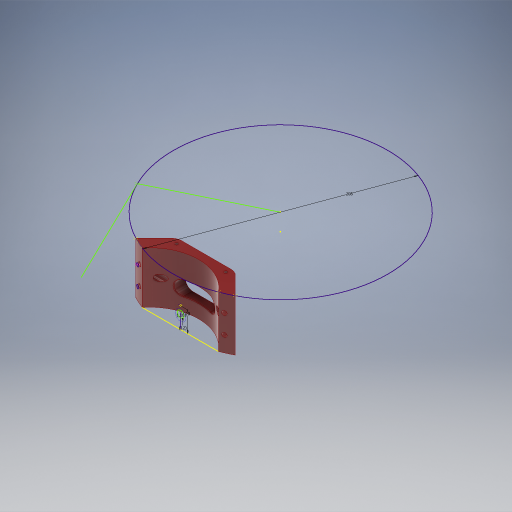
# Autodesk Inventor part: catch_v2
Saved by Autodesk Inventor 2023 (Build 270158000, 158)
## iProperties
Created: 2024-11-02
Part Number: catch_v2
Material: Полиэтилен, низкая плотность
Document SubType Name: Sheet Metal
Designer: Ivan
Density: 0.579707 g/cm^3
Appearance: Типовые
Mass: 30 g
Surface Area: 146.87 cm^2
Volume: 51.7503 cm^3
Sheet Metal Rule: По умолчанию
Author: Ivan
Autodesk Inventor part; units mm, degrees
ref_plane "YZ Plane" through (0, 0, 0) normal (1, 0, 0) x (0, 1, 0)
ref_plane "XZ Plane" through (0, 0, 0) normal (0, 1, 0) x (-1, 0, 0)
ref_plane "XY Plane" through (0, 0, 0) normal (0, 0, 1) x (1, 0, 0)
derived "floor_v2.ipt"
sketch "Эскиз2" plane through (0, 0, 0) normal (0, 1, 0) x (1, 0, 0)
  circle A0 centre (0, 0) radius 107.5
  circle A1 centre (0, 0) radius 104
  line L0 (0, 0) -> (104, 0) construction
  line L1 (0, 0) -> (0, -104) construction
  line L2 (0, 0) -> (-104, 0) construction
  line L3 (0, 0) -> (0, 104) construction
  line L4 (104, 0) -> (0, -104) construction
  line L5 (0, 104) -> (-104, 0) construction
  line L6 (0, -104) -> (-104, 0) construction
  line L7 (104, 0) -> (0, 104) construction
  line L8 (0, 0) -> (-73.5391, -73.5391) construction
  line L9 (0, 0) -> (73.5391, -73.5391) construction
  line L10 (0, 0) -> (73.5391, 73.5391) construction
  line L11 (0, 0) -> (-73.5391, 73.5391) construction
  line L12 (-38.4471, -82.2877) -> (-82.2877, -38.4471)
  line L13 (-38.4471, -82.2877) -> (-48.2758, -92.1165)
  line L14 (-82.2877, -38.4471) -> (-92.1165, -48.2758)
  line L15 (92.1165, -48.2758) -> (82.2877, -38.4471)
  line L16 (82.2877, -38.4471) -> (38.4471, -82.2877)
  line L17 (38.4471, -82.2877) -> (48.2758, -92.1165)
  line L18 (48.2758, 92.1165) -> (38.4471, 82.2877)
  line L19 (38.4471, 82.2877) -> (82.2877, 38.4471)
  line L20 (82.2877, 38.4471) -> (92.1165, 48.2758)
  line L21 (-48.2758, 92.1165) -> (-38.4471, 82.2877)
  line L22 (-38.4471, 82.2877) -> (-82.2877, 38.4471)
  line L23 (-82.2877, 38.4471) -> (-92.1165, 48.2758)
  line L24 (0, -107.5) -> (0, -79.5) construction
  circle A2 centre (0, -116.5) radius 37 construction
  circle A3 centre (0, -127) radius 47.5
  line L25 (0, 107.5) -> (0, 79.5) construction
  circle A4 centre (0, 127) radius 47.5
  line L26 (-92.1165, 48.2758) -> (-94.7051, 50.8645)
  line L27 (-48.2758, 92.1165) -> (-50.8645, 94.7051)
  line L28 (48.2758, 92.1165) -> (50.8645, 94.7051)
  line L29 (92.1165, 48.2758) -> (94.7051, 50.8645)
  line L30 (92.1165, -48.2758) -> (94.7051, -50.8645)
  line L31 (48.2758, -92.1165) -> (50.8645, -94.7051)
  line L32 (-92.1165, -48.2758) -> (-94.7051, -50.8645)
  line L33 (-48.2758, -92.1165) -> (-50.8645, -94.7051)
  point P0 (-52, -52)
  point P1 (-52, 52)
  point P2 (52, 52)
  point P3 (52, -52)
  point P4 (-60.3674, -60.3674)
  point P5 (60.3674, -60.3674)
  point P6 (60.3674, 60.3674)
  point P7 (-60.3674, 60.3674)
  point P8 (-36.9892, -97.1998)
  point P9 (36.9892, -97.1998)
  point P10 (36.9892, 97.1998)
  point P11 (-36.9892, 97.1998)
sketch "Эскиз3" plane through (0, 2, 0) normal (0, -1, 0) x (-1, 0, 0)
  line L0 (33.8509, 77.6915) -> (77.6915, 33.8509) construction
  line L1 (55.7712, 55.7712) -> (0, 0) construction
  line L2 (44.4575, 67.0849) -> (67.0849, 44.4575) construction
  circle A0 centre (44.4575, 67.0849) radius 1.5
  circle A1 centre (67.0849, 44.4575) radius 1.5
  line L3 (28.3991, 51.0265) -> (51.0265, 28.3991) construction
  circle A2 centre (28.3991, 51.0265) radius 1.5
  circle A3 centre (51.0265, 28.3991) radius 1.5
  line L4 (44.4575, -67.0849) -> (67.0849, -44.4575) construction
  line L5 (28.3991, -51.0265) -> (51.0265, -28.3991) construction
  line L6 (55.7712, -55.7712) -> (0, 0) construction
  line L7 (-55.7712, -55.7712) -> (0, 0) construction
  line L8 (-28.3991, -51.0265) -> (-51.0265, -28.3991) construction
  line L9 (-44.4575, -67.0849) -> (-67.0849, -44.4575) construction
  line L10 (-55.7712, 55.7712) -> (0, 0) construction
  line L11 (-51.0265, 28.3991) -> (-28.3991, 51.0265) construction
  line L12 (-67.0849, 44.4575) -> (-44.4575, 67.0849) construction
  circle A4 centre (-44.4575, 67.0849) radius 1.5
  circle A5 centre (-67.0849, 44.4575) radius 1.5
  circle A6 centre (-28.3991, 51.0265) radius 1.5
  circle A7 centre (-51.0265, 28.3991) radius 1.5
  circle A8 centre (-44.4575, -67.0849) radius 1.5
  circle A9 centre (-67.0849, -44.4575) radius 1.5
  circle A10 centre (-51.0265, -28.3991) radius 1.5
  circle A11 centre (-28.3991, -51.0265) radius 1.5
  circle A12 centre (44.4575, -67.0849) radius 1.5
  circle A13 centre (28.3991, -51.0265) radius 1.5
  circle A14 centre (51.0265, -28.3991) radius 1.5
  circle A15 centre (67.0849, -44.4575) radius 1.5
  line L13 (-38.4471, -82.2877) -> (-82.2877, -38.4471)
  line L14 (82.2877, -38.4471) -> (38.4471, -82.2877)
  line L15 (38.4471, 82.2877) -> (82.2877, 38.4471)
  line L16 (-82.2877, 38.4471) -> (-38.4471, 82.2877)
  line L17 (82.2877, 38.4471) -> (92.1165, 48.2758)
  point P0 (39.7128, 39.7128)
  point P1 (-39.7128, -39.7128)
  point P2 (39.7128, -39.7128)
  point P3 (-39.7128, 39.7128)
  point P4 (-40.1306, -40.1306)
sketch "Эскиз6" plane through (0, 2, 0) normal (0, -1, 0) x (-1, 0, 0)
  arc A0 (36.9892, -97.1998) -> (-36.9892, -97.1998) centre (0, -127) ccw
  arc A1 (-36.9892, 97.1998) -> (36.9892, 97.1998) centre (0, 127) ccw
  point P0 (-0.0301, 154.5629)
  point P1 (-0.0412, -154.5628)
sketch "Эскиз8" plane through (0, 2, 0) normal (0, 1, 0) x (1, 0, 0)
  arc A0 (-48.2758, -92.1165) -> (-36.9892, -97.1998) centre (0, 0) ccw
  arc A1 (36.9892, -97.1998) -> (48.2758, -92.1165) centre (0, 0) ccw
  arc A2 (36.9892, -97.1998) -> (-36.9892, -97.1998) centre (0, -127) ccw
  circle A3 centre (0, -127) radius 55.4164 construction
  circle A4 centre (-23.8556, -76.9811) radius 1.5
  circle A5 centre (23.8556, -76.9811) radius 1.5
  circle A6 centre (-28.3991, -51.0265) radius 1.5 construction
  circle A7 centre (-51.0265, -28.3991) radius 1.5 construction
  circle A8 centre (-67.0849, -44.4575) radius 1.5 construction
  circle A9 centre (-44.4575, -67.0849) radius 1.5 construction
  circle A10 centre (-51.0265, -28.3991) radius 1.5 construction
  line L0 (-51.0265, -28.3991) -> (-28.3991, -51.0265) construction
  line L1 (-67.0849, -44.4575) -> (-44.4575, -67.0849) construction
  line L2 (-55.7712, -55.7712) -> (-39.7128, -39.7128) construction
  line L3 (-50.4184, -50.4184) -> (-23.8556, -76.9811) construction
  circle A11 centre (67.0849, -44.4575) radius 1.5 construction
  circle A12 centre (44.4575, -67.0849) radius 1.5 construction
  line L4 (44.4575, -67.0849) -> (67.0849, -44.4575) construction
  arc A13 (-92.1165, 48.2758) -> (-92.1165, -48.2758) centre (0, 0) ccw construction
  line L5 (-104, 0) -> (104, 0) construction
  arc A14 (92.1165, -48.2758) -> (92.1165, 48.2758) centre (0, 0) ccw construction
  circle A15 centre (-23.8556, 76.9811) radius 1.5
  circle A16 centre (23.8556, 76.9811) radius 1.5
  point P0 (-44.5136, -93.9922)
  point P1 (-104, 0)
sketch "Эскиз5" plane through (0, 0, 0) normal (0, 1, 0) x (-1, 0, 0)
  arc A0 (-36.9892, 97.1998) -> (36.9892, 97.1998) centre (0, 127) ccw projected
  circle A1 centre (0, 0) radius 104 projected
  line L0 (38.4471, 82.2877) -> (48.2758, 92.1165) projected
  line L1 (-38.4471, 82.2877) -> (-48.2758, 92.1165) projected
  line L2 (38.4471, 82.2877) -> (28.1405, 71.9811)
  line L3 (-38.4471, 82.2877) -> (-28.1405, 71.9811)
  line L4 (28.1405, 71.9811) -> (-28.1405, 71.9811)
  line L5 (82.2877, 38.4471) -> (38.4471, 82.2877) projected
  circle A2 centre (23.8556, 76.9811) radius 1.5 projected
  circle A3 centre (-23.8556, 76.9811) radius 1.5 projected
  circle A4 centre (23.8556, 76.9811) radius 5 construction
  circle A5 centre (-23.8556, 76.9811) radius 5 construction
  dimension "d3" = 10
  constraints: 6 end point, 2 centre point, 2 coincident, 2 collinear, 2 tangent, 1 horizontal, 1 perpendicular
  measures "d3" diameter of A5
extrude "Выдавливание1" add sketch "Эскиз5" along normal blind 50 contours A0 A1 L0 L2 L4 L3 L1 | A2 | A3
ref_plane "РабПлоскость2" through (0, 0, 43.8406) normal (-1, 0, 0) x (0, 1, 0)
sketch "Эскиз9" plane through (0, 50, 0) normal (0, 1, 0) x (1, 0, 0)
  circle A0 centre (-23.8556, -76.9811) radius 1.5 projected
  circle A1 centre (23.8556, -76.9811) radius 1.5 projected
  point P0 (0, 0)
hole "Отверстие1" at (-23.8556, 50, 76.9811) at (23.8556, 50, 76.9811) direction (0, -1, 0) diameter 3.2 depth 7
hole "Отверстие2" at (-23.8556, 0, 76.9811) at (23.8556, 0, 76.9811) direction (0, 1, 0) diameter 3.2 depth 7
fillet "Сопряжение1" radius 10 2 edges at (-28.1405, 25, 71.9811) (28.1405, 25, 71.9811)
ref_plane "РабПлоскость1" through (-36.9892, 50, 97.1998) normal (-1, 0, 0) x (0, 1, 0)
sketch "Эскиз10" plane through (-36.9892, 50, 97.1998) normal (-1, 0, 0) x (0, 1, 0)
  line L0 (-50, 0) -> (0, 0) projected
  line L1 (-25, 0) -> (-25, -14.2479)
  circle A0 centre (-25, 8.49) radius 3.1
  line L2 (0, 17.6998) -> (0, 0) projected
  line L3 (0, 17.6998) -> (-25, 17.6998)
  line L4 (0, 17.6998) -> (-50, 17.6998) projected
  point P0 (-50, 97.1998)
  dimension "d21" = 6.2
  dimension "d54" = 8.49
  constraints: 4 end point, 2 midpoint, 2 point on line, 1 centre point, 1 perpendicular
  measures "d21" diameter of A0
  measures "d54" distance from line of L0 A0.centre
extrude "Выдавливание2" cut sketch "Эскиз10" along normal through all both and the other way through all
mirror "Зеркальное отражение1" about plane through (0, 0, 43.8406) normal (-1, 0, 0) of "Выдавливание2"
ref_plane "РабПлоскость3" through (0, 25, 0) normal (0, 1, 0) x (1, 0, 0)
sketch "Эскиз13" plane through (48.2758, 0, 92.1165) normal (0.7071068, 0, -0.7071068) x (-0.7071068, 0, -0.7071068)
  line L0 (-186.6107, 25) -> (379.5577, 25) projected
  line L1 (24.3335, 50) -> (24.3335, 0) projected
  point P0 (99.2724, 0)
sketch "Эскиз17" plane through (0, 50, 0) normal (0, 1, 0) x (1, 0, 0)
  line L0 (-31.0695, -74.9101) -> (-48.2758, -92.1165) projected
  arc A0 (-48.2758, -92.1165) -> (-36.9892, -97.1998) centre (0, 0) ccw projected
  line L1 (-40.9045, -84.7452) -> (-40.9045, -95.6181)
  line L2 (-36.9892, -79.5) -> (-36.9892, -97.1998) projected
  arc A1 (36.9892, -97.1998) -> (-36.9892, -97.1998) centre (0, -127) ccw projected
  line L3 (-24.2555, -86.1598) -> (-42.3192, -86.1598) projected
  line L4 (-31.9045, -91.8098) -> (-47.9692, -91.8098) projected
  dimension "d55" = 9
  constraints: 2 end point, 1 parallel, 1 point on circle, 1 point on line
  measures "d55" distance from line of L1 L4.start
ref_plane "РабПлоскость5" through (-40.9045, 50, 95.6181) normal (-1, 0, 0) x (0, 1, 0)
sketch "Эскиз18" plane through (-40.9045, 50, 95.6181) normal (-1, 0, 0) x (0, 1, 0)
  circle A0 centre (-25, 6.9083) radius 3.1 projected
  circle A1 centre (-25, 6.9083) radius 3.1
  point P0 (-50, 95.6181)
  dimension "d56" = 6.2
  constraints: 2 coincident, 1 centre point
  measures "d56" diameter of A1
extrude "Выдавливание7" cut sketch "Эскиз18" along normal blind 13
mirror "Зеркальное отражение3" about plane through (0, 0, 43.8406) normal (-1, 0, 0) of "Выдавливание7"
ref_plane "РабПлоскость7" through (36.9892, 50, 97.1998) normal (-0.6749966, 0, -0.7378208) x (-0.7378208, 0, 0.6749966)
ref_plane "РабПлоскость6" through (93.533, -2, 45.4705) normal (-0.6749966, 0, -0.7378208) x (-0.7378208, 0, 0.6749966)
sketch "Эскиз19" plane through (36.9892, 50, 97.1998) normal (-0.6749966, 0, -0.7378208) x (-0.7378208, 0, 0.6749966)
  spline S0 degree 3 poles (-7.7154, -10.575) (-7.7154, -10.6506) (-7.71, -10.7286) (-7.6802, -10.9332) (-7.6461, -11.0604) (-7.5316, -11.3409) (-7.4453, -11.4844) (-7.2515, -11.7106) (-7.1586, -11.7978) (-6.897, -11.9868) (-6.7118, -12.075) (-6.3289, -12.1741) (-6.1042, -12.1918) (-5.7271, -12.1319) (-5.5774, -12.0862) (-5.2959, -11.9511) (-5.167, -11.8652) (-4.8829, -11.6031) (-4.7406, -11.4053) (-4.5272, -10.8834) (-4.4982, -10.5576) (-4.6133, -10.0143) (-4.7143, -9.7949) (-4.9564, -9.4713) (-5.0835, -9.3525) (-5.3442, -9.1705) (-5.4898, -9.0986) (-5.9017, -8.9666) (-6.1741, -8.9581) (-6.6389, -9.0429) (-6.8486, -9.1334) (-7.1761, -9.3613) (-7.2993, -9.4844) (-7.4685, -9.7101) (-7.5294, -9.8144) (-7.6283, -10.0387) (-7.6645, -10.1561) (-7.7063, -10.3754) (-7.7154, -10.4772) (-7.7154, -10.575) knots 0 0 0 0 0.030068 0.030068 0.078176 0.078176 0.140718 0.140718 0.183173 0.183173 0.246087 0.246087 0.309229 0.309229 0.349946 0.349946 0.390663 0.390663 0.445235 0.445235 0.518423 0.518423 0.571305 0.571305 0.612987 0.612987 0.654495 0.654495 0.727263 0.727263 0.799075 0.799075 0.857025 0.857025 0.901749 0.901749 0.946474 0.946474 0.985357 0.985357 0.985357 0.985357 weights 1 1 1 1 1 1 1 1 1 1 1 1 1 1 1 1 1 1 1 1 1 1 1 1 1 1 1 1 1 1 1 1 1 1 1 1 1 1 1 1 projected
  spline S1 degree 3 poles (-7.7154, -40.575) (-7.7154, -40.6506) (-7.71, -40.7286) (-7.6802, -40.9332) (-7.6461, -41.0604) (-7.5316, -41.3409) (-7.4453, -41.4844) (-7.2515, -41.7106) (-7.1586, -41.7978) (-6.897, -41.9868) (-6.7118, -42.075) (-6.3289, -42.1741) (-6.1042, -42.1918) (-5.7271, -42.1319) (-5.5774, -42.0862) (-5.2959, -41.9511) (-5.167, -41.8652) (-4.8829, -41.6031) (-4.7406, -41.4053) (-4.5272, -40.8834) (-4.4982, -40.5576) (-4.6133, -40.0143) (-4.7143, -39.7949) (-4.9564, -39.4713) (-5.0835, -39.3525) (-5.3442, -39.1705) (-5.4898, -39.0986) (-5.9017, -38.9666) (-6.1741, -38.9581) (-6.6389, -39.0429) (-6.8486, -39.1334) (-7.1761, -39.3613) (-7.2993, -39.4844) (-7.4685, -39.7101) (-7.5294, -39.8144) (-7.6283, -40.0387) (-7.6645, -40.1561) (-7.7063, -40.3754) (-7.7154, -40.4772) (-7.7154, -40.575) knots 0 0 0 0 0.030068 0.030068 0.078176 0.078176 0.140718 0.140718 0.183173 0.183173 0.246087 0.246087 0.309229 0.309229 0.349946 0.349946 0.390663 0.390663 0.445235 0.445235 0.518423 0.518423 0.571305 0.571305 0.612987 0.612987 0.654495 0.654495 0.727263 0.727263 0.799075 0.799075 0.857025 0.857025 0.901749 0.901749 0.946474 0.946474 0.985357 0.985357 0.985357 0.985357 weights 1 1 1 1 1 1 1 1 1 1 1 1 1 1 1 1 1 1 1 1 1 1 1 1 1 1 1 1 1 1 1 1 1 1 1 1 1 1 1 1 projected
  point P0 (-38.3182, -50)
  point P1 (-7.7154, -10.575)
  point P2 (-7.7154, -40.575)
ref_plane "РабПлоскость8" through (-36.9892, 50, 97.1998) normal (0, 0, 1) x (0, -1, 0)
sketch "Эскиз21" plane through (-36.9892, 50, 97.1998) normal (0, 0, 1) x (0, -1, 0)
  ellipse E0 centre (38, 37.1664) end of major axis (32.9, 37.1664) minor radius 5.1 construction
  line L0 (50, 0) -> (50, 73.9783) projected
  line L1 (38, 37.1664) -> (50, 37.1664)
  circle A0 centre (36.839, 37.1664) radius 3.1623
  point P0 (50, 36.9892)
  point P1 (30, 37.1664)
  dimension "d75" = 12
  dimension "d76" = 1.161
  dimension "d93" = 20
  constraints: 3 point on line, 2 end point, 1 centre point, 1 perpendicular, 3 other
  measures "d75" distance of L1.start L1.end
  measures "d76" distance of L1.start A0.centre
  measures "d93" distance from line of point (30, 37.166) L0
hole "Отверстие5" at (0.1772, 20, 97.1998) direction (0, 0, -1) diameter 13.5 end through all
sketch "Эскиз23" plane through (0, 50, 0) normal (0, 1, 0) x (1, 0, 0)
  circle A0 centre (0, 0) radius 104
  line L0 (-93.5502, -45.4353) -> (-42.0243, -151.5258)
  line L1 (-93.5502, -45.4353) -> (0, 0)
  arc A1 (-48.2758, -92.1165) -> (-36.9892, -97.1998) centre (0, 0) ccw projected
  point P0 (48.2758, -92.1165)
  point P1 (36.9892, -97.1998)
  dimension "d77" = 208
  constraints: 4 end point, 2 point on circle, 1 centre point, 1 concentric, 1 point on line, 1 tangent
  measures "d77" diameter of A0
ref_plane "РабПлоскость9" through (-41.7508, 33.5167, 97.0505) normal (0, 1, 0) x (1, 0, 0)
sketch "Эскиз24" plane through (-41.7508, 33.5167, 97.0505) normal (0, 1, 0) x (1, 0, 0)
  point P0 (41.7508, 97.0505)
  point P1 (0, 0)
ref_plane "РабПлоскость10" through (-41.7508, 33.5167, 97.0505) normal (-0.3951802, 0, 0.9186036) x (0, -1, 0)
sketch "Эскиз25" plane through (-41.7508, 33.5167, 97.0505) normal (-0.3951802, 0, 0.9186036) x (0, -1, 0)
  spline S0 degree 3 poles (-1.6, 0) (-1.6, 0.0991) (-1.5907, 0.2016) (-1.5393, 0.4672) (-1.4807, 0.6292) (-1.2922, 0.9686) (-1.154, 1.1294) (-0.8735, 1.3476) (-0.7502, 1.4203) (-0.4207, 1.5587) (-0.2036, 1.6) (0.2036, 1.6) (0.4207, 1.5587) (0.8178, 1.392) (0.9977, 1.2668) (1.321, 0.9392) (1.4676, 0.6925) (1.6159, 0.1629) (1.6205, -0.1058) (1.5045, -0.5857) (1.408, -0.7897) (1.1869, -1.0839) (1.0823, -1.1886) (0.8337, -1.3744) (0.6918, -1.4515) (0.3653, -1.569) (0.1774, -1.6) (-0.0952, -1.6) (-0.1934, -1.5914) (-0.5126, -1.5323) (-0.7306, -1.4409) (-0.9964, -1.2559) (-1.0718, -1.1917) (-1.2278, -1.0337) (-1.3094, -0.9291) (-1.4884, -0.6265) (-1.5607, -0.4119) (-1.5959, -0.1327) (-1.6, -0.0656) (-1.6, 0) knots 0.72325 0.72325 0.72325 0.72325 0.753388 0.753388 0.801609 0.801609 0.864296 0.864296 0.904063 0.904063 0.964334 0.964334 1.024605 1.024605 1.084875 1.084875 1.162686 1.162686 1.242644 1.242644 1.304846 1.304846 1.349406 1.349406 1.393966 1.393966 1.446501 1.446501 1.474685 1.474685 1.538426 1.538426 1.567042 1.567042 1.605057 1.605057 1.667632 1.667632 1.687584 1.687584 1.687584 1.687584 weights 1 1 1 1 1 1 1 1 1 1 1 1 1 1 1 1 1 1 1 1 1 1 1 1 1 1 1 1 1 1 1 1 1 1 1 1 1 1 1 1
  spline S1 degree 3 poles (16.7833, 0) (16.7833, 0.0991) (16.7927, 0.2016) (16.844, 0.4672) (16.9026, 0.6292) (17.0911, 0.9686) (17.2293, 1.1294) (17.5098, 1.3476) (17.6331, 1.4203) (17.9627, 1.5587) (18.1798, 1.6) (18.5869, 1.6) (18.804, 1.5587) (19.2011, 1.392) (19.3811, 1.2668) (19.7044, 0.9392) (19.851, 0.6925) (19.9992, 0.1629) (20.0038, -0.1058) (19.8879, -0.5857) (19.7913, -0.7897) (19.5702, -1.0839) (19.4656, -1.1886) (19.217, -1.3744) (19.0751, -1.4515) (18.7486, -1.569) (18.5608, -1.6) (18.2881, -1.6) (18.1899, -1.5914) (17.8707, -1.5323) (17.6527, -1.4409) (17.387, -1.2559) (17.3115, -1.1917) (17.1555, -1.0337) (17.074, -0.9291) (16.895, -0.6265) (16.8226, -0.4119) (16.7874, -0.1327) (16.7833, -0.0656) (16.7833, 0) knots 0.72325 0.72325 0.72325 0.72325 0.753388 0.753388 0.801609 0.801609 0.864296 0.864296 0.904063 0.904063 0.964334 0.964334 1.024605 1.024605 1.084875 1.084875 1.162686 1.162686 1.242644 1.242644 1.304846 1.304846 1.349406 1.349406 1.393966 1.393966 1.446501 1.446501 1.474685 1.474685 1.538426 1.538426 1.567042 1.567042 1.605057 1.605057 1.667632 1.667632 1.687584 1.687584 1.687584 1.687584 weights 1 1 1 1 1 1 1 1 1 1 1 1 1 1 1 1 1 1 1 1 1 1 1 1 1 1 1 1 1 1 1 1 1 1 1 1 1 1 1 1
  constraints: 4 other
sketch "Эскиз26" plane through (-41.7508, 33.5167, 97.0505) normal (-0.3951802, 0, 0.9186036) x (0, -1, 0)
  spline S0 degree 3 poles (-1.6, 0) (-1.6, 0.0991) (-1.5907, 0.2016) (-1.5393, 0.4672) (-1.4807, 0.6292) (-1.2922, 0.9686) (-1.154, 1.1294) (-0.8735, 1.3476) (-0.7502, 1.4203) (-0.4207, 1.5587) (-0.2036, 1.6) (0.2036, 1.6) (0.4207, 1.5587) (0.8178, 1.392) (0.9977, 1.2668) (1.321, 0.9392) (1.4676, 0.6925) (1.6159, 0.1629) (1.6205, -0.1058) (1.5045, -0.5857) (1.408, -0.7897) (1.1869, -1.0839) (1.0823, -1.1886) (0.8337, -1.3744) (0.6918, -1.4515) (0.3653, -1.569) (0.1774, -1.6) (-0.0952, -1.6) (-0.1934, -1.5914) (-0.5126, -1.5323) (-0.7306, -1.4409) (-0.9964, -1.2559) (-1.0718, -1.1917) (-1.2278, -1.0337) (-1.3094, -0.9291) (-1.4884, -0.6265) (-1.5607, -0.4119) (-1.5959, -0.1327) (-1.6, -0.0656) (-1.6, 0) knots 0.72325 0.72325 0.72325 0.72325 0.753388 0.753388 0.801609 0.801609 0.864296 0.864296 0.904063 0.904063 0.964334 0.964334 1.024605 1.024605 1.084875 1.084875 1.162686 1.162686 1.242644 1.242644 1.304846 1.304846 1.349406 1.349406 1.393966 1.393966 1.446501 1.446501 1.474685 1.474685 1.538426 1.538426 1.567042 1.567042 1.605057 1.605057 1.667632 1.667632 1.687584 1.687584 1.687584 1.687584 weights 1 1 1 1 1 1 1 1 1 1 1 1 1 1 1 1 1 1 1 1 1 1 1 1 1 1 1 1 1 1 1 1 1 1 1 1 1 1 1 1 construction
  circle A0 centre (0, 0) radius 2
  line L0 (33.5167, 4.4331) -> (-16.4833, 4.4331) projected
  line L1 (8.5167, 4.4331) -> (8.5167, -8) construction
  line L2 (-16.4833, -67.9804) -> (-16.4833, 21.2763) projected
  line L3 (33.5167, 4.4331) -> (33.5167, -7.9438) projected
  spline S1 degree 3 poles (16.7833, 0) (16.7833, 0.0991) (16.7927, 0.2016) (16.844, 0.4672) (16.9026, 0.6292) (17.0911, 0.9686) (17.2293, 1.1294) (17.5098, 1.3476) (17.6331, 1.4203) (17.9627, 1.5587) (18.1798, 1.6) (18.5869, 1.6) (18.804, 1.5587) (19.2011, 1.392) (19.3811, 1.2668) (19.7044, 0.9392) (19.851, 0.6925) (19.9992, 0.1629) (20.0038, -0.1058) (19.8879, -0.5857) (19.7913, -0.7897) (19.5702, -1.0839) (19.4656, -1.1886) (19.217, -1.3744) (19.0751, -1.4515) (18.7486, -1.569) (18.5608, -1.6) (18.2881, -1.6) (18.1899, -1.5914) (17.8707, -1.5323) (17.6527, -1.4409) (17.387, -1.2559) (17.3115, -1.1917) (17.1555, -1.0337) (17.074, -0.9291) (16.895, -0.6265) (16.8226, -0.4119) (16.7874, -0.1327) (16.7833, -0.0656) (16.7833, 0) knots 0.72325 0.72325 0.72325 0.72325 0.753388 0.753388 0.801609 0.801609 0.864296 0.864296 0.904063 0.904063 0.964334 0.964334 1.024605 1.024605 1.084875 1.084875 1.162686 1.162686 1.242644 1.242644 1.304846 1.304846 1.349406 1.349406 1.393966 1.393966 1.446501 1.446501 1.474685 1.474685 1.538426 1.538426 1.567042 1.567042 1.605057 1.605057 1.667632 1.667632 1.687584 1.687584 1.687584 1.687584 weights 1 1 1 1 1 1 1 1 1 1 1 1 1 1 1 1 1 1 1 1 1 1 1 1 1 1 1 1 1 1 1 1 1 1 1 1 1 1 1 1 projected
  circle A1 centre (18.3832, -0.0001) radius 1.5999
  line L4 (18.3832, -0.0001) -> (16.7833, -0.0001) construction
  line L5 (18.3832, -0.0001) -> (19.1831, -1.3856) construction
  line L6 (18.3832, -0.0001) -> (19.1831, 1.3854) construction
  line L7 (33.5167, 1.0625) -> (-16.4833, 1.0625) projected
  circle A2 centre (18.3832, -0.0001) radius 2
  point P0 (33.5167, 0)
  point P1 (-1.6, 0)
  dimension "d86" = 4
  dimension "d87" = 50
  dimension "d88" = 25
  dimension "d89" = 120
  dimension "d90" = 120
  constraints: 8 end point, 4 coincident, 3 centre point, 3 point on circle, 1 equal radius, 1 horizontal, 1 midpoint, 1 vertical, 4 other
  measures "d86" diameter of A0
  measures "d87" distance between parallel lines of L3 L2
  measures "d88" distance between parallel lines of L1 L2
  measures "d89" angle of L4 L5
  measures "d90" angle of L6 L4
extrude "Выдавливание10" cut sketch "Эскиз26" against normal blind 8.15 contours A0 L7 | L7 A0 | A2 L7 S1 | L7 S1 A2 | L7 S1 | S1 L7
ref_plane "РабПлоскость11" through (0, 0, 43.8406) normal (-1, 0, 0) x (0, 1, 0)
mirror "Зеркальное отражение5" about plane through (0, 0, 43.8406) normal (-1, 0, 0) of "Выдавливание10"
sketch "Эскиз27" plane through (-36.9892, 50, 97.1998) normal (0, 0, 1) x (0, -1, 0)
  line L0 (23.25, 17.1664) -> (36.75, 17.1664)
  line L1 (36.75, 17.1664) -> (36.75, 57.1664)
  line L2 (36.75, 57.1664) -> (23.25, 57.1664)
  line L3 (23.25, 57.1664) -> (23.25, 17.1664)
  line L4 (23.25, 23.9164) -> (36.75, 23.9164)
  line L5 (36.75, 50.4164) -> (23.25, 50.4164)
  arc A0 (23.25, 23.9164) -> (36.75, 23.9164) centre (30, 23.9164) ccw
  arc A1 (36.75, 50.4164) -> (23.25, 50.4164) centre (30, 50.4164) ccw
  line L6 (38, 37.1664) -> (50, 37.1664) projected
  line L7 (50, 12.9908) -> (50, 5.9197) projected
  line L8 (0, 5.9197) -> (0, 12.9908) projected
  line L9 (0, 12.9908) -> (50, 12.9908) projected
  line L10 (50, 68.0586) -> (50, 60.9876) projected
  line L11 (0, 60.9876) -> (0, 68.0586) projected
  line L12 (50, 60.9876) -> (0, 60.9876) projected
  point P0 (50, 36.9892)
  point P1 (30, 57.1664)
  point P2 (30, 17.1664)
  point P3 (36.75, 37.1664)
  point P4 (30, 57.1664)
  point P5 (30, 17.1664)
  dimension "d94" = 40
  constraints: 12 end point, 6 midpoint, 6 point on circle, 5 point on line, 3 perpendicular, 2 centre point, 2 parallel, 2 vertical, 1 coincident, 1 equal radius, 1 horizontal, 1 other
  measures "d94" distance of point (30, 57.166) point (30, 17.166)
extrude "Выдавливание11" cut sketch "Эскиз27" against normal through all contours A0 L4 | L3 L5 L1 L4 | A1 L5
chamfer "Фаска2" distance 0.5 angle 45 4 edges at (0.1845, 13.25, 79.5004) (-19.8228, 19.9982, 83.834) (0.1845, 26.75, 79.5004) (20.1772, 20.0019, 83.9985)
chamfer "Фаска3" distance 0.5 angle 45 4 edges at (-19.8228, 20, 71.9811) (0.1772, 13.25, 71.9811) (20.1772, 20, 71.9811) (0.1772, 26.75, 71.9811)
equation "\"d3\" = d2"
equation "\"d88\" = 0.5 * d87"
equation "\"Радиус_гибки\" = Толщина"
equation "\"Ширина_просечки\" = Толщина"
equation "\"Глубина_просечки\" = 0.5 * Толщина"
equation "\"Размер_просечки\" = 4 * Толщина"
equation "\"Мин_остаток\" = 2 * Толщина"
equation "\"Радиус_перехода\" = Радиус_гибки"
equation "\"Радиус_Якоби\" = Радиус_гибки"
equation "\"Размер_зазора\" = Толщина"
equation "\"d2\" = 10"
equation "\"Толщина\" = 3.048"
